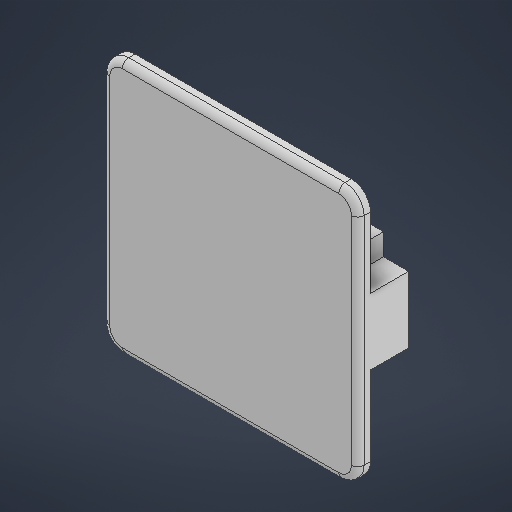
# Autodesk Inventor part: затычка
Saved by Autodesk Inventor 2025 (Build 290162000, 162)
## iProperties
Created: 2024-12-14
Part Number: затычка
Material: Типовые
Document SubType Name: Modeling
Designer: Phantom
Density: 1 g/cm^3
Appearance: По умолчанию
Author: Phantom
Autodesk Inventor part; units mm, degrees
ref_plane "YZ Plane" through (0, 0, 0) normal (1, 0, 0) x (0, 1, 0)
ref_plane "XZ Plane" through (0, 0, 0) normal (0, 1, 0) x (-1, 0, 0)
ref_plane "XY Plane" through (0, 0, 0) normal (0, 0, 1) x (1, 0, 0)
sketch "Эскиз1" plane through (0, 0, 0) normal (0, 0, 1) x (1, 0, 0)
  circle A0 centre (0, 0) radius 2.5
  circle A1 centre (7.6, 7.6) radius 1.5
  circle A2 centre (-7.6, 7.6) radius 1.5
  circle A3 centre (-7.6, -7.6) radius 1.5
  circle A4 centre (7.6, -7.6) radius 1.5
  arc A5 (-8.5, 10) -> (-10, 8.5) centre (-8.5, 8.5) ccw
  line L0 (-8.5, 10) -> (8.5, 10)
  line L1 (-10, -8.5) -> (-10, 8.5)
  line L2 (-10, -8.5) -> (-10, -3.95)
  arc A6 (-10, -8.5) -> (-8.5, -10) centre (-8.5, -8.5) ccw
  line L3 (-3.95, -10) -> (-8.5, -10)
  line L4 (8.5, -10) -> (-8.5, -10)
  arc A7 (8.5, -10) -> (10, -8.5) centre (8.5, -8.5) ccw
  line L5 (10, -3.95) -> (10, -8.5)
  line L6 (10, 8.5) -> (10, -8.5)
  arc A8 (10, 8.5) -> (8.5, 10) centre (8.5, 8.5) ccw
  line L7 (3.95, 10) -> (8.5, 10)
  constraints: 16 end point, 9 centre point, 8 point on circle, 1 coincident
extrude "Выдавливание1" add sketch "Эскиз1" along normal blind 1 contours A0 | A1 | A2 | A3 | A4 | L0 A8 L6 L5 A7 L4 L3 A6 L1 A5
fillet "Сопряжение1" radius 0.5 8 edges at (-9.5607, -9.5607, 1) (0, -10, 1) (9.5607, -9.5607, 1) (10, -6.225, 1) (9.5607, 9.5607, 1) (6.225, 10, 1) (-9.5607, 9.5607, 1) (-10, -6.225, 1)
sketch "Эскиз2" plane through (0, 0, 0) normal (0, 0, -1) x (-1, 0, 0)
  circle A0 centre (0, 0) radius 2.5
  constraints: 1 centre point, 1 coincident
extrude "Выдавливание2" add sketch "Эскиз2" along normal blind 3
fillet "Сопряжение2" radius 1 1 edges at (2.5, 0, -3)
sketch "Эскиз3" plane through (0, 0, 0) normal (0, 0, -1) x (-1, 0, 0)
  line L0 (-10, -8.5) -> (-10, 8.5) projected
  line L1 (0, 0) -> (0, -8.5)
  arc A0 (6.2205, -3.7242) -> (6.8074, -3.9673) centre (6.8074, -3.1373) ccw
  line L2 (8.0499, -3.9673) -> (6.8074, -3.9673)
  line L3 (8.0267, -3.2811) -> (8.0407, -3.2952)
  line L4 (4.6459, 0.629) -> (4.6459, 2.1594)
  arc A1 (5.1321, 3.3332) -> (4.6459, 2.1594) centre (6.3059, 2.1594) ccw
  line L5 (6.8074, 4.6647) -> (8.0267, 4.6647)
  line L6 (6.2205, -3.7242) -> (5.1321, -2.6359)
  arc A2 (4.6459, -1.4621) -> (5.1321, -2.6359) centre (6.3059, -1.4621) ccw
  arc A3 (6.8074, 4.6647) -> (6.2205, 4.4216) centre (6.8074, 3.8347) ccw
  line L7 (5.1321, 3.3332) -> (6.2205, 4.4216)
  arc A4 (4.6459, 0.0684) -> (4.6431, 0.1025) centre (4.4384, 0.0684) ccw
  line L8 (4.6459, -1.4621) -> (4.6459, 0.629)
  arc A5 (4.6431, 0.5948) -> (4.6459, 0.629) centre (4.4384, 0.629) ccw
  line L9 (8.0499, -3.9673) -> (8.0267, -2.2602)
  line L10 (7.9913, 0.3493) -> (4.6459, 0.3493)
  line L11 (9.9996, 5.5485) -> (10, 5.5489)
  line L12 (8.0267, 2.9588) -> (8.0267, 4.6647)
  line L13 (8.0267, 2.9588) -> (10, 2.9588)
  line L14 (10, 8.5) -> (10, -8.5) projected
  line L15 (8.0267, -2.2602) -> (10, -2.2602)
  arc A6 (-6.8074, -3.9673) -> (-6.2205, -3.7242) centre (-6.8074, -3.1373) ccw
  line L16 (-8.0499, -3.9673) -> (-6.8074, -3.9673)
  line L17 (-8.0267, -3.2811) -> (-8.0407, -3.2952)
  line L18 (-6.2205, -3.7242) -> (-5.1321, -2.6359)
  arc A7 (-5.1321, -2.6359) -> (-4.6459, -1.4621) centre (-6.3059, -1.4621) ccw
  line L19 (-8.0499, -3.9673) -> (-8.0267, -2.2602)
  arc A8 (-4.6431, 0.1025) -> (-4.6459, 0.0684) centre (-4.4384, 0.0684) ccw
  line L20 (-4.6459, 0.629) -> (-4.6459, 2.1594)
  arc A9 (-4.6459, 2.1594) -> (-5.1321, 3.3332) centre (-6.3059, 2.1594) ccw
  line L21 (-6.8074, 4.6647) -> (-8.0267, 4.6647)
  line L22 (-7.9913, 0.3493) -> (-4.6459, 0.3493)
  arc A10 (-4.6459, 0.629) -> (-4.6431, 0.5948) centre (-4.4384, 0.629) ccw
  line L23 (-4.6459, -1.4621) -> (-4.6459, 0.629)
  line L24 (-9.9996, 5.5485) -> (-10, 5.5489)
  line L25 (-8.0267, 2.9588) -> (-8.0267, 4.6647)
  line L26 (-5.1321, 3.3332) -> (-6.2205, 4.4216)
  arc A11 (-6.2205, 4.4216) -> (-6.8074, 4.6647) centre (-6.8074, 3.8347) ccw
  line L27 (-8.0267, 2.9588) -> (-10, 2.9588)
  line L28 (-8.0267, -2.2602) -> (-10, -2.2602)
  point P0 (10, -4.8504)
  point P1 (-10, -4.8504)
  constraints: 54 end point, 32 symmetric about line, 24 point on circle, 12 centre point, 10 point on line, 2 horizontal, 1 vertical, 6 other
extrude "Выдавливание3" add sketch "Эскиз3" along normal blind 3
